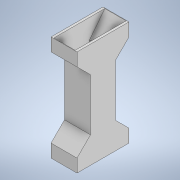
# Autodesk Inventor part: Bone_Cover
Saved by Autodesk Inventor 2022 (Build 260153000, 153)
## iProperties
Created: 2022-01-22
Part Number: Bone_Cover
Material: Generic
Document SubType Name: Modeling
Designer: Mlees
Density: 1 g/cm^3
Appearance: Default
Author: Mlees
Autodesk Inventor part; units mm, degrees
ref_plane "YZ Plane" through (0, 0, 0) normal (1, 0, 0) x (0, 1, 0)
sketch "Sketch1" plane through (0, 0, 0) normal (0, 1, 0) x (-1, 0, 0)
  line L0 (0, 0) -> (34, 0)
  line L1 (34, 0) -> (34, -80)
  line L2 (34, -80) -> (0, -80)
  line L3 (0, -80) -> (0, 0)
  dimension "d0" = 34
  dimension "d1" = 80
  constraints: 8 end point, 2 parallel, 1 horizontal, 1 perpendicular
  measures "d0" distance of L1.end L2.end
  measures "d1" distance of L0.end L1.end
extrude "Extrusion1" add sketch "Sketch1" along normal blind 30
ref_plane "Work Plane1" through (-17, 0, 0) normal (1, 0, 0) x (0, 0, -1)
sketch "Sketch2" plane through (-17, 0, 0) normal (1, 0, 0) x (0, 0, -1)
  line L0 (80, 30) -> (0, 30) projected
  line L1 (40, 30) -> (27.3, 30)
  line L2 (40, 30) -> (52.7, 30)
  line L3 (52.7, 30) -> (55.7, 30)
  line L4 (80, 0) -> (80, 30) projected
  line L5 (80, 0) -> (79.25, 0)
  line L6 (80, 0) -> (0, 0) projected
  line L7 (79.25, 0) -> (55.7, 30)
  line L8 (27.3, 30) -> (24.3, 30)
  line L9 (0, 0) -> (0.75, 0)
  line L10 (0.75, 0) -> (24.3, 30)
  line L11 (0.75, 0) -> (79.25, 0)
  dimension "d4" = 12.7
  dimension "d5" = 12.7
  dimension "d6" = 3
  dimension "d7" = 0.75
  dimension "d8" = 3
  dimension "d9" = 0.75
  constraints: 18 end point, 6 point on line, 1 collinear, 1 midpoint
  measures "d4" distance of L1.start L1.end
  measures "d5" distance of L1.start L2.end
  measures "d6" distance of L2.end L3.end
  measures "d7" distance of L4.start L5.end
  measures "d8" distance of L1.end L8.end
  measures "d9" distance of L6.end L9.end
extrude "Extrusion2" cut sketch "Sketch2" along normal mid plane 32.8 contours L7 L6 L10 L0
sketch "Sketch3" plane through (-34, 0, -80) normal (-1, 0, 0) x (0, 0, 1)
  line L0 (80, 30) -> (0, 30) projected
  line L1 (0, 0) -> (80, 0) projected
  line L2 (0, 30) -> (80, 30)
  line L3 (80, 30) -> (80, 0)
  line L4 (80, 0) -> (0, 0)
  line L5 (0, 0) -> (0, 30)
  constraints: 8 end point, 2 parallel, 1 horizontal, 1 perpendicular
extrude "Extrusion3" add sketch "Sketch3" along normal blind 3
sketch "Sketch4" plane through (0, 0, 0) normal (1, 0, 0) x (0, 0, -1)
  line L0 (0, 0) -> (0, 30) projected
  line L1 (0, 0) -> (80, 0) projected
  line L2 (0, 30) -> (80, 30)
  line L3 (80, 30) -> (80, 0)
  line L4 (80, 0) -> (0, 0)
  line L5 (0, 0) -> (0, 30)
  constraints: 8 end point, 2 parallel, 1 horizontal, 1 perpendicular
extrude "Extrusion4" add sketch "Sketch4" along normal blind 3
sketch "Sketch5" plane through (3, 0, 0) normal (1, 0, 0) x (0, 0, -1)
  line L0 (0, 30) -> (80, 30) projected
  line L1 (0, 30) -> (0, 20)
  line L2 (0, 0) -> (0, 30) projected
  line L3 (0, 30) -> (10, 30)
  line L4 (10, 30) -> (0, 20)
  line L5 (80, 30) -> (80, 0) projected
  line L6 (80, 30) -> (80, 20)
  line L7 (80, 30) -> (70, 30)
  line L8 (70, 30) -> (80, 20)
  dimension "d16" = 10
  dimension "d17" = 10
  dimension "d18" = 10
  constraints: 12 end point, 4 point on line
  measures "d16" distance of L0.start L1.end
  measures "d17" distance of L0.start L3.end
  measures "d18" distance of L0.end L7.end
extrude "Extrusion5" cut sketch "Sketch5" against normal through all
sketch "Sketch6" plane through (0, 30, 0) normal (0, 1, 0) x (1, 0, 0)
  line L0 (-0.6, 24.3) -> (-33.4, 24.3) projected
  line L1 (-0.6, 55.7) -> (-0.6, 24.3) projected
  line L2 (-33.4, 24.3) -> (-0.6, 24.3)
  line L3 (-0.6, 24.3) -> (-0.6, 55.7)
  line L4 (-0.6, 55.7) -> (-33.4, 55.7)
  line L5 (-33.4, 55.7) -> (-33.4, 24.3)
  line L6 (-37, 20.7) -> (3, 20.7)
  line L7 (3, 20.7) -> (3, 59.3)
  line L8 (3, 59.3) -> (-37, 59.3)
  line L9 (-37, 59.3) -> (-37, 20.7)
  point P0 (0, 0)
  dimension "d21" = 3.6
  constraints: 16 end point, 4 parallel, 2 perpendicular, 1 horizontal, 3 other
  measures "d21" distance between parallel lines of L5 L9
extrude "Extrusion6" add sketch "Sketch6" along normal blind 76.2
sketch "Sketch7" plane through (3, 0, 0) normal (1, 0, 0) x (0, 0, -1)
  line L0 (20.7, 30) -> (10, 30) projected
  line L1 (10, 30) -> (20.7, 40.7)
  line L2 (20.7, 30) -> (20.7, 106.2) projected
  line L3 (10, 30) -> (25.1321, 30) construction
  line L4 (20.7, 40.7) -> (20.7, 30)
  line L5 (20.7, 30) -> (10, 30)
  line L6 (70, 30) -> (59.3, 30) projected
  line L7 (70, 30) -> (59.3, 40.7)
  line L8 (59.3, 30) -> (59.3, 106.2) projected
  line L9 (59.3, 40.7) -> (59.3, 30)
  line L10 (70, 30) -> (80, 20) projected
  line L11 (59.3, 30) -> (70, 30)
  point P0 (0, 0)
  dimension "d24" = 45
  constraints: 14 end point, 3 perpendicular, 2 collinear, 2 point on line, 1 equal length, 1 horizontal
  measures "d24" angle of L3 L1
extrude "Extrusion7" add sketch "Sketch7" against normal up to surface (40 mm away)
ref_plane "Work Plane2" through (0, 80.8, 0) normal (0, 1, 0) x (1, 0, 0)
mirror "Mirror1" about plane through (0, 80.8, 0) normal (0, 1, 0)
body "Solid1"
